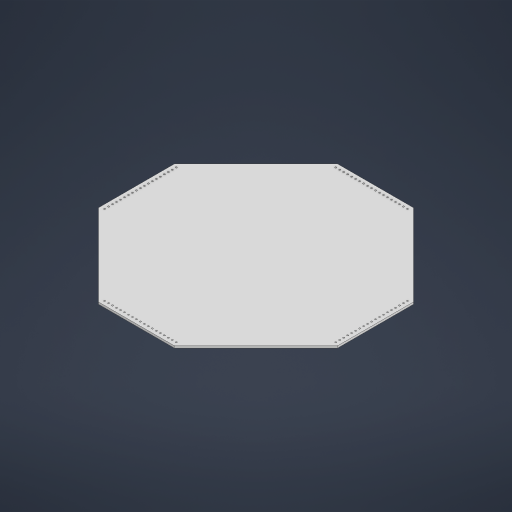
# Autodesk Inventor part: Belly Pan
Saved by Autodesk Inventor 2024.3 (Build 283343000, 343)
## iProperties
Created: 2024-11-27
Part Number: Belly Pan
Material: Generic
Document SubType Name: Modeling
Designer: kaito
Density: 1 g/cm^3
Appearance: Default
Author: kaito
Autodesk Inventor part; units mm, degrees
ref_plane "YZ Plane" through (0, 0, 0) normal (1, 0, 0) x (0, 1, 0)
ref_plane "XZ Plane" through (0, 0, 0) normal (0, 1, 0) x (-1, 0, 0)
ref_plane "XY Plane" through (0, 0, 0) normal (0, 0, 1) x (1, 0, 0)
sketch "Sketch1" plane through (0, 0, 0) normal (0, 1, 0) x (-1, 0, 0)
  line L0 (0, 0) -> (762, 0) construction
  line L1 (762, 0) -> (762, -762)
  line L2 (762, -762) -> (0, -762)
  line L3 (762, -260.35) -> (736.6, -260.35) construction
  line L4 (736.6, -260.35) -> (736.6, -501.65) construction
  line L5 (736.6, -501.65) -> (762, -501.65) construction
  line L6 (762, -501.65) -> (762, -260.35) construction
  line L7 (501.65, 0) -> (260.35, 0)
  line L8 (260.35, 0) -> (260.35, -25.4) construction
  line L9 (260.35, -25.4) -> (501.65, -25.4) construction
  line L10 (501.65, -25.4) -> (501.65, 0) construction
  line L11 (501.65, -762) -> (260.35, -762) construction
  line L12 (260.35, -762) -> (260.35, -736.6) construction
  line L13 (260.35, -736.6) -> (501.65, -736.6) construction
  line L14 (501.65, -736.6) -> (501.65, -762) construction
  line L15 (0, 0) -> (0, -762)
  line L16 (0, -260.35) -> (25.4, -260.35) construction
  line L17 (25.4, -260.35) -> (25.4, -501.65) construction
  line L18 (25.4, -501.65) -> (0, -501.65) construction
  line L19 (0, -501.65) -> (0, -260.35) construction
  line L20 (260.35, 0) -> (0, -260.35)
  line L21 (501.65, 0) -> (762, -260.35)
  line L22 (762, -501.65) -> (501.65, -762)
  line L23 (0, -501.65) -> (260.35, -762)
  circle A0 centre (12.7, -266.7) radius 2.4892
  circle A1 centre (12.7, -279.4) radius 2.4892
  line L24 (25.4, -273.05) -> (25.4, -514.35) construction
  circle A2 centre (12.7, -292.1) radius 2.4892
  line L25 (25.4, -285.75) -> (25.4, -527.05) construction
  circle A3 centre (12.7, -304.8) radius 2.4892
  line L26 (25.4, -298.45) -> (25.4, -539.75) construction
  circle A4 centre (12.7, -317.5) radius 2.4892
  line L27 (25.4, -311.15) -> (25.4, -552.45) construction
  circle A5 centre (12.7, -330.2) radius 2.4892
  line L28 (25.4, -323.85) -> (25.4, -565.15) construction
  circle A6 centre (12.7, -342.9) radius 2.4892
  line L29 (25.4, -336.55) -> (25.4, -577.85) construction
  circle A7 centre (12.7, -355.6) radius 2.4892
  line L30 (25.4, -349.25) -> (25.4, -590.55) construction
  circle A8 centre (12.7, -368.3) radius 2.4892
  line L31 (25.4, -361.95) -> (25.4, -603.25) construction
  circle A9 centre (12.7, -381) radius 2.4892
  line L32 (25.4, -374.65) -> (25.4, -615.95) construction
  circle A10 centre (12.7, -393.7) radius 2.4892
  line L33 (25.4, -387.35) -> (25.4, -628.65) construction
  circle A11 centre (12.7, -406.4) radius 2.4892
  line L34 (25.4, -400.05) -> (25.4, -641.35) construction
  circle A12 centre (12.7, -419.1) radius 2.4892
  line L35 (25.4, -412.75) -> (25.4, -654.05) construction
  circle A13 centre (12.7, -431.8) radius 2.4892
  line L36 (25.4, -425.45) -> (25.4, -666.75) construction
  circle A14 centre (12.7, -444.5) radius 2.4892
  line L37 (25.4, -438.15) -> (25.4, -679.45) construction
  circle A15 centre (12.7, -457.2) radius 2.4892
  line L38 (25.4, -450.85) -> (25.4, -692.15) construction
  circle A16 centre (12.7, -469.9) radius 2.4892
  line L39 (25.4, -463.55) -> (25.4, -704.85) construction
  circle A17 centre (12.7, -482.6) radius 2.4892
  line L40 (25.4, -476.25) -> (25.4, -717.55) construction
  circle A18 centre (12.7, -495.3) radius 2.4892
  line L41 (25.4, -488.95) -> (25.4, -730.25) construction
  circle A19 centre (495.3, -12.7) radius 2.4892
  circle A20 centre (482.6, -12.7) radius 2.4892
  circle A21 centre (469.9, -12.7) radius 2.4892
  circle A22 centre (457.2, -12.7) radius 2.4892
  circle A23 centre (444.5, -12.7) radius 2.4892
  circle A24 centre (431.8, -12.7) radius 2.4892
  circle A25 centre (419.1, -12.7) radius 2.4892
  circle A26 centre (406.4, -12.7) radius 2.4892
  circle A27 centre (393.7, -12.7) radius 2.4892
  circle A28 centre (381, -12.7) radius 2.4892
  circle A29 centre (368.3, -12.7) radius 2.4892
  circle A30 centre (355.6, -12.7) radius 2.4892
  circle A31 centre (342.9, -12.7) radius 2.4892
  circle A32 centre (330.2, -12.7) radius 2.4892
  circle A33 centre (317.5, -12.7) radius 2.4892
  circle A34 centre (304.8, -12.7) radius 2.4892
  circle A35 centre (292.1, -12.7) radius 2.4892
  circle A36 centre (279.4, -12.7) radius 2.4892
  circle A37 centre (266.7, -12.7) radius 2.4892
  circle A38 centre (749.3, -266.7) radius 2.4892
  circle A39 centre (749.3, -279.4) radius 2.4892
  circle A40 centre (749.3, -292.1) radius 2.4892
  circle A41 centre (749.3, -304.8) radius 2.4892
  circle A42 centre (749.3, -317.5) radius 2.4892
  circle A43 centre (749.3, -330.2) radius 2.4892
  circle A44 centre (749.3, -342.9) radius 2.4892
  circle A45 centre (749.3, -355.6) radius 2.4892
  circle A46 centre (749.3, -368.3) radius 2.4892
  circle A47 centre (749.3, -381) radius 2.4892
  circle A48 centre (749.3, -393.7) radius 2.4892
  circle A49 centre (749.3, -406.4) radius 2.4892
  circle A50 centre (749.3, -419.1) radius 2.4892
  circle A51 centre (749.3, -431.8) radius 2.4892
  circle A52 centre (749.3, -444.5) radius 2.4892
  circle A53 centre (749.3, -457.2) radius 2.4892
  circle A54 centre (749.3, -469.9) radius 2.4892
  circle A55 centre (749.3, -482.6) radius 2.4892
  circle A56 centre (749.3, -495.3) radius 2.4892
  circle A57 centre (495.3, -749.3) radius 2.4892
  circle A58 centre (482.6, -749.3) radius 2.4892
  circle A59 centre (469.9, -749.3) radius 2.4892
  circle A60 centre (457.2, -749.3) radius 2.4892
  circle A61 centre (444.5, -749.3) radius 2.4892
  circle A62 centre (431.8, -749.3) radius 2.4892
  circle A63 centre (419.1, -749.3) radius 2.4892
  circle A64 centre (406.4, -749.3) radius 2.4892
  circle A65 centre (393.7, -749.3) radius 2.4892
  circle A66 centre (381, -749.3) radius 2.4892
  circle A67 centre (368.3, -749.3) radius 2.4892
  circle A68 centre (355.6, -749.3) radius 2.4892
  circle A69 centre (342.9, -749.3) radius 2.4892
  circle A70 centre (330.2, -749.3) radius 2.4892
  circle A71 centre (317.5, -749.3) radius 2.4892
  circle A72 centre (304.8, -749.3) radius 2.4892
  circle A73 centre (292.1, -749.3) radius 2.4892
  circle A74 centre (279.4, -749.3) radius 2.4892
  circle A75 centre (266.7, -749.3) radius 2.4892
  point P0 (736.6, -381)
  point P1 (381, -25.4)
  point P2 (381, 0)
  point P3 (381, -736.6)
  point P4 (381, -762)
  point P5 (25.4, -381)
  point P6 (0, -381)
  point P7 (762, -381)
  point P8 (25.4, -393.7)
  point P9 (25.4, -406.4)
  point P10 (25.4, -419.1)
  point P11 (25.4, -431.8)
  point P12 (25.4, -444.5)
  point P13 (25.4, -457.2)
  point P14 (25.4, -469.9)
  point P15 (25.4, -482.6)
  point P16 (25.4, -495.3)
  point P17 (25.4, -508)
  point P18 (25.4, -520.7)
  point P19 (25.4, -533.4)
  point P20 (25.4, -546.1)
  point P21 (25.4, -558.8)
  point P22 (25.4, -571.5)
  point P23 (25.4, -584.2)
  point P24 (25.4, -596.9)
  point P25 (12.7, -260.35)
  point P26 (12.7, -501.65)
  point P27 (25.4, -609.6)
  point P28 (501.65, -12.7)
  point P29 (749.3, -260.35)
  point P30 (501.65, -749.3)
  dimension "d0" = 762
  dimension "d1" = 762
  dimension "d4" = 25.4
  dimension "d5" = 241.3
  dimension "d6" = 25.4
  dimension "d7" = 241.3
  dimension "d8" = 25.4
  dimension "d9" = 25.4
  dimension "d10" = 241.3
  dimension "d11" = 241.3
  dimension "d12" = 4.9784
  dimension "d15" = 12.7
  dimension "d20" = 6.35
  dimension "d21" = 19.05
  dimension "d22" = 4.9784
  dimension "d23" = 6.35
  dimension "d26" = 12.7
  dimension "d31" = 4.9784
  dimension "d32" = 6.35
  dimension "d35" = 12.7
  dimension "d40" = 4.9784
  dimension "d41" = 6.35
  dimension "d44" = 12.7
  constraints: 84 end point, 76 centre point, 13 midpoint, 9 parallel, 7 horizontal, 5 perpendicular, 4 horizontal alignment, 4 point on line, 3 vertical, 3 vertical alignment, 1 collinear, 215 other
  measures "d0" distance of L1.end L2.end
  measures "d1" distance of L0.end L1.end
  measures "d4" distance of L5.end L4.end
  measures "d5" distance of L9.end L8.end
  measures "d6" distance of L8.end L7.end
  measures "d7" distance of L12.end L13.end
  measures "d8" distance of L11.end L12.end
  measures "d9" distance of L17.end L18.end
  measures "d10" distance of L16.end L17.end
  measures "d11" distance of L3.end L4.end
  measures "d12" diameter of A0
  measures "d15" distance of A0.centre A1.centre
  measures "d20" distance of A0.centre point (12.7, -260.35)
  measures "d21" distance of point (12.7, -501.65) A17.centre
  measures "d22" diameter of A19
  measures "d23" distance from line of L10 A19.centre
  measures "d26" distance of A19.centre A20.centre
  measures "d31" diameter of A38
  measures "d32" distance of point (749.3, -260.35) A38.centre
  measures "d35" distance of A38.centre A39.centre
  measures "d40" diameter of A57
  measures "d41" distance of A57.centre point (501.65, -749.3)
  measures "d44" distance of A57.centre A58.centre
extrude "Extrusion1" add sketch "Sketch1" along normal blind 6.35 contours L1 L22 L2 L23 L15 L20 L7 L21
body "Solid1"
